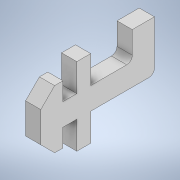
# Autodesk Inventor part: cable holder
Saved by Autodesk Inventor 2020 (Build 240168000, 168)
## iProperties
Created: 2020-01-06
Part Number: cable holder
Material: Générique
Document SubType Name: Modeling
Designer: damien
Density: 1 g/cm^3
Appearance: Par défaut
Author: damien
Autodesk Inventor part; units mm, degrees
ref_plane "YZ Plane" through (0, 0, 0) normal (1, 0, 0) x (0, 1, 0)
ref_plane "XZ Plane" through (0, 0, 0) normal (0, 1, 0) x (-1, 0, 0)
ref_plane "XY Plane" through (0, 0, 0) normal (0, 0, 1) x (1, 0, 0)
sketch "Esquisse1" plane through (0, 0, 0) normal (1, 0, 0) x (0, 1, 0)
  line L0 (-5.5, 0) -> (5.5, 0)
  line L1 (10.5, -8) -> (4, -8)
  line L2 (4, -8) -> (4, -13)
  line L3 (4, -13) -> (14, -13)
  line L4 (14, -13) -> (14, -18)
  line L5 (14, -18) -> (4, -18)
  line L6 (-10.5, -8) -> (-4, -8)
  line L7 (-4, -8) -> (-4, -13)
  line L8 (-4, -13) -> (-14, -13)
  line L9 (-14, -13) -> (-14, -18)
  line L10 (-14, -18) -> (-4, -18)
  line L11 (4, -18) -> (4, -33)
  line L12 (-4, -18) -> (-4, -41)
  line L13 (5.5, 0) -> (10.5, -5)
  line L14 (10.5, -5) -> (10.5, -8)
  line L15 (-5.5, 0) -> (-10.5, -5)
  line L16 (-10.5, -5) -> (-10.5, -8)
  line L17 (14, -33) -> (14, -41)
  line L18 (4, -33) -> (14, -33)
  line L19 (14, -41) -> (-4, -41)
  point P0 (0, 0)
  point P1 (0, 0)
  dimension "d0" = 8
  dimension "d1" = 8
  dimension "d2" = 3
  dimension "d3" = 10
  dimension "d6" = 5
  dimension "d7" = 5
  dimension "d10" = 21
  dimension "d11" = 45
  dimension "d14" = 10
  dimension "d15" = 8
  dimension "d16" = 15
  dimension "d17" = 28
  dimension "d18" = 28
  constraints: 41 end point, 8 perpendicular, 6 equal length, 4 vertical, 3 horizontal, 3 parallel, 2 point on line, 1 coincident, 1 collinear, 1 midpoint
  measures "d0" distance between parallel lines of L7 L2
  measures "d1" distance between parallel lines of L1 L0
  measures "d2" distance of L13.end L1.start
  measures "d3" distance of L4.end L5.end
  measures "d6" distance between parallel lines of L5 L3
  measures "d7" distance of L1.end L2.end
  measures "d10" distance between parallel lines of L16 L14
  measures "d11" angle of L16 L15
  measures "d14" distance between parallel lines of L11 L17
  measures "d15" distance between parallel lines of L19 L18
  measures "d16" distance between parallel lines of L18 L5
  measures "d17" distance between parallel lines of L19 L3
  measures "d18" distance between parallel lines of L4 L9
extrude "Extrusion1" add sketch "Esquisse1" along normal blind 5.5
fillet "Congé1" radius 2 2 edges at (2.75, -4, -41) (2.75, 4, -33)
